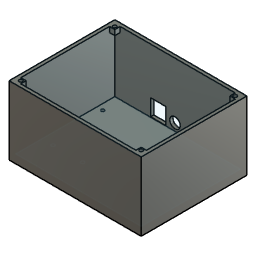
Arduino_Housing_v7 (Autodesk Fusion 360 design; units mm, degrees)
Autodesk Fusion 360 part; units mm, degrees
sketch "Sketch1" plane through (0, 0, 0) normal (0, 1, 0) x (1, 0, 0)
  line L0 (0, 0) -> (125, 0)
  line L1 (125, 0) -> (125, -100)
  line L2 (125, -100) -> (0, -100)
  line L3 (0, -100) -> (0, 0)
  dimension "d1" = 125
  dimension "d2" = 100
  constraint horizontal L0
  constraint vertical L1
  constraint horizontal L2
  constraint vertical L3
  constraint coincident L0.start L3.end
  measures "d1" distance of L0.start L0.end
  measures "d2" distance of L0.start L2.end
extrude "Extrude1" add sketch "Sketch1" along normal blind 5
sketch "Sketch2" plane through (0, 5, 0) normal (0, 1, 0) x (-1, 0, 0)
  line L0 (0, 100) -> (-125, 100)
  line L1 (-125, 100) -> (-125, 0)
  line L2 (-125, 0) -> (0, 0)
  line L3 (0, 0) -> (0, 100)
  line L4 (-122, 3) -> (-3, 3)
  line L5 (-3, 3) -> (-3, 97)
  line L6 (-3, 97) -> (-122, 97)
  line L7 (-122, 97) -> (-122, 3)
  line L8 (-6, 6) -> (-59.3, 6)
  line L9 (-59.3, 6) -> (-59.3, 74.6)
  line L10 (-59.3, 74.6) -> (-6, 74.6)
  line L11 (-6, 74.6) -> (-6, 6)
  line L12 (-59.3, 6) -> (-52.3, 6)
  line L13 (-6, 6) -> (-37, 6)
  line L14 (-37, 3) -> (-52, 3)
  line L15 (-52, 3) -> (-52, 0)
  line L16 (-52, 0) -> (-37, 0)
  line L17 (-37, 0) -> (-37, 3)
  line L18 (-6, 6) -> (-6, 19.97)
  circle A0 centre (-8.54, 19.97) radius 1.5
  line L19 (-6, 6) -> (-6, 72.04)
  circle A1 centre (-13.62, 72.04) radius 1.65
  circle A2 centre (-41.56, 72.04) radius 1.65
  line L20 (-119, 6) -> (-64, 6)
  line L21 (-64, 6) -> (-64, 90)
  line L22 (-64, 90) -> (-119, 90)
  line L23 (-119, 90) -> (-119, 6)
  dimension "d9" = 53.3
  dimension "d10" = 68.6
  dimension "d11" = 7
  dimension "d12" = 31
  dimension "d13" = 13.97
  dimension "d14" = 2.54
  dimension "d15" = 3
  dimension "d16" = 66.04
  dimension "d17" = 7.62
  dimension "d18" = 35.56
  dimension "d19" = 3.3
  dimension "d20" = 3.3
  dimension "d21" = 55
  dimension "d22" = 84
  constraint horizontal L4
  constraint vertical L5
  constraint horizontal L6
  constraint vertical L7
  constraint horizontal L8
  constraint vertical L9
  constraint horizontal L10
  constraint vertical L11
  constraint perpendicular L9 L12
  constraint perpendicular L11 L13
  constraint horizontal L14
  constraint vertical L15
  constraint horizontal L16
  constraint vertical L17
  constraint coincident L2 L15.end
  constraint coincident L4 L14.start
  constraint perpendicular L13 L18
  constraint perpendicular L13 L19
  constraint horizontal L20
  constraint vertical L21
  constraint horizontal L22
  constraint vertical L23
  measures "d9" distance of L8.start L8.end
  measures "d10" distance of L8.start L10.end
  measures "d11" distance of L8.end L12.end
  measures "d12" distance of L8.start L13.end
  measures "d13" distance of L8.start L18.end
  measures "d14" distance of L18.end A0.centre
  measures "d15" diameter of A0
  measures "d16" distance of L8.start L19.end
  measures "d17" distance of L19.end A1.centre
  measures "d18" distance of L19.end A2.centre
  measures "d19" diameter of A1
  measures "d20" diameter of A2
  measures "d21" distance of L20.start L20.end
  measures "d22" distance of L20.start L22.end
extrude "Extrude2" cut sketch "Sketch2" against normal blind 5 contours A0 | A1 | A2
sketch "Sketch3" plane through (0, 5, 0) normal (0, 1, 0) x (-1, 0, 0)
  circle A0 centre (-8.54, 19.97) radius 1.5
  circle A1 centre (-13.62, 72.04) radius 1.65
  circle A2 centre (-41.56, 72.04) radius 1.65
  line L0 (0, 100) -> (-125, 100)
  line L1 (-125, 100) -> (-125, 0)
  line L2 (-125, 0) -> (0, 0)
  line L3 (0, 0) -> (0, 100)
  line L4 (-3, 3) -> (-123.5, 3)
  line L5 (-123.5, 3) -> (-123.5, 98.5)
  line L6 (-123.5, 98.5) -> (-3, 98.5)
  line L7 (-3, 98.5) -> (-3, 3)
  line L8 (-6, 6) -> (-59.3, 6)
  line L9 (-59.3, 6) -> (-59.3, 74.6)
  line L10 (-59.3, 74.6) -> (-6, 74.6)
  line L11 (-6, 74.6) -> (-6, 6)
  line L12 (-6, 6) -> (-37, 6)
  line L13 (-59.3, 6) -> (-51.3, 6)
  line L14 (-37, 3) -> (-51.3, 3)
  line L15 (-51.3, 3) -> (-51.3, 0)
  line L16 (-51.3, 0) -> (-37, 0)
  line L17 (-37, 0) -> (-37, 3)
  dimension "d25" = 53.3
  dimension "d26" = 68.6
  dimension "d27" = 31
  dimension "d28" = 8
  constraint horizontal L4
  constraint vertical L5
  constraint horizontal L6
  constraint vertical L7
  constraint horizontal L8
  constraint vertical L9
  constraint horizontal L10
  constraint vertical L11
  constraint perpendicular L11 L12
  constraint perpendicular L9 L13
  constraint horizontal L14
  constraint vertical L15
  constraint horizontal L16
  constraint vertical L17
  constraint coincident L2 L15.end
  constraint coincident L4 L14.start
  measures "d25" distance of L8.start L8.end
  measures "d26" distance of L8.start L10.end
  measures "d27" distance of L8.start L12.end
  measures "d28" distance of L8.end L13.end
extrude "Extrude3" add sketch "Sketch3" along normal blind 1 contours L0 L1 L2 L3 L4 L5 L6 L7 L15 L17
sketch "Sketch4" plane through (0, 0, 0) normal (0, -1, 0) x (1, 0, 0)
  circle A0 centre (8.54, 19.97) radius 1.5
  circle A1 centre (13.62, 72.04) radius 1.65
  circle A2 centre (41.56, 72.04) radius 1.65
  line L0 (125, 100) -> (0, 100)
  line L1 (0, 100) -> (0, 0)
  line L2 (0, 0) -> (125, 0)
  line L3 (125, 0) -> (125, 100)
  circle A3 centre (8.54, 19.97) radius 3.5
  circle A4 centre (13.62, 72.04) radius 3.5
  circle A5 centre (41.56, 72.04) radius 3.5
  dimension "d31" = 7
  dimension "d32" = 7
  dimension "d33" = 7
  constraint concentric A0 A3
  constraint concentric A1 A4
  constraint concentric A2 A5
  measures "d31" diameter of A3
  measures "d32" diameter of A4
  measures "d33" diameter of A5
extrude "Extrude4" cut sketch "Sketch4" against normal blind 2.5 contours A3 | A4 | A5
extrude "Extrude5" add 1 faces at (1, 6, 34.3333) along direction (0, 1, 0) blind 17
sketch "Sketch5" plane through (0, 5, 0) normal (0, 1, 0) x (-1, 0, 0)
  line L0 (-51.3, 3) -> (-51.3, 0)
  line L1 (-51.3, 0) -> (-37, 0)
  line L2 (-37, 0) -> (-37, 3)
  line L3 (-37, 3) -> (-3, 3)
  line L4 (-3, 3) -> (-3, 98.5)
  line L5 (-3, 98.5) -> (-123.5, 98.5)
  line L6 (-123.5, 98.5) -> (-123.5, 3)
  line L7 (-123.5, 3) -> (-51.3, 3)
  circle A0 centre (-8.54, 19.97) radius 1.5
  circle A1 centre (-13.62, 72.04) radius 1.65
  circle A2 centre (-41.56, 72.04) radius 1.65
  line L8 (-51.3, 3) -> (-37, 3)
  line L9 (-37, 3) -> (-37, 0)
  line L10 (-37, 0) -> (-51.3, 0)
  line L11 (-51.3, 0) -> (-51.3, 3)
  constraint horizontal L8
  constraint vertical L9
  constraint horizontal L10
  constraint vertical L11
  constraint coincident L1.end L2.start
  constraint coincident L0.start L7.end
extrude "Extrude6" add sketch "Sketch5" along normal blind 0.4 contours L0 L1 L2 L8 L9 L10 L11
extrude "Extrude7" cut 1 faces at (1, 23, 34.3333) along direction (0, -1, 0) blind 2
sketch "Sketch6" plane through (0, 21, 0) normal (0, 1, 0) x (-1, 0, 0)
  line L0 (0, 0) -> (0, 100)
  line L1 (0, 100) -> (-125, 100)
  line L2 (-125, 100) -> (-125, 0)
  line L3 (-125, 0) -> (-51.3, 0)
  line L4 (-51.3, 0) -> (-51.3, 3)
  line L5 (-51.3, 3) -> (-123.5, 3)
  line L6 (-123.5, 3) -> (-123.5, 98.5)
  line L7 (-123.5, 98.5) -> (-3, 98.5)
  line L8 (-3, 98.5) -> (-3, 3)
  line L9 (-3, 3) -> (-37, 3)
  line L10 (-37, 3) -> (-37, 0)
  line L11 (-37, 0) -> (0, 0)
  line L12 (-37, 0) -> (-51.3, 0)
  line L13 (-51.3, 0) -> (-51.3, 3)
  line L14 (-51.3, 3) -> (-37, 3)
  line L15 (-37, 3) -> (-37, 0)
  constraint horizontal L12
  constraint vertical L13
  constraint horizontal L14
  constraint vertical L15
  constraint coincident L4.end L5.start
  constraint coincident L10.end L11.start
extrude "Extrude8" add sketch "Sketch6" along normal blind 44 contours L0 L1 L2 L3 L4 L5 L6 L7 L8 L9 L10 L11 L13 L15 | L4 L10 L12 L13 L14 L15
sketch "Sketch7" plane through (0, 0, 3) normal (0, 0, 1) x (1, 0, 0)
  line L0 (3, 65) -> (3, 5)
  line L1 (3, 5) -> (123.5, 5)
  line L2 (123.5, 5) -> (123.5, 65)
  line L3 (123.5, 65) -> (3, 65)
  line L4 (37, 21) -> (51.3, 21)
  line L5 (51.3, 21) -> (51.3, 5.4)
  line L6 (51.3, 5.4) -> (37, 5.4)
  line L7 (37, 5.4) -> (37, 21)
  circle A0 centre (60, 12) radius 5
  dimension "d44" = 10
  measures "d44" diameter of A0
extrude "Extrude9" cut sketch "Sketch7" against normal blind 3 contours A0
extrude "Extrude10" add 1 faces at (43.1667, 45, 98.5) along direction (0, 0, -1) blind 1.5
extrude "Extrude11" add 1 faces at (123.5, 25, 34.3333) along direction (-1, 0, 0) blind 1.5
sketch "Sketch8" plane through (0, 5, 0) normal (0, 1, 0) x (-1, 0, 0)
  line L0 (-122, 97) -> (-122, 3)
  line L1 (-122, 3) -> (-3, 3)
  line L2 (-3, 3) -> (-3, 97)
  line L3 (-3, 97) -> (-122, 97)
  circle A0 centre (-41.56, 72.04) radius 1.65
  circle A1 centre (-13.62, 72.04) radius 1.65
  circle A2 centre (-8.54, 19.97) radius 1.5
sketch "Sketch9" plane through (0, 65, 0) normal (0, 1, 0) x (-1, 0, 0)
  line L0 (-3, 3) -> (-122, 3)
  line L1 (-122, 3) -> (-122, 97)
  line L2 (-122, 97) -> (-3, 97)
  line L3 (-3, 97) -> (-3, 3)
  line L4 (0, 0) -> (0, 100)
  line L5 (0, 100) -> (-125, 100)
  line L6 (-125, 100) -> (-125, 0)
  line L7 (-125, 0) -> (0, 0)
  line L8 (-122, 97) -> (-112, 97)
  line L9 (-112, 97) -> (-112, 87)
  line L10 (-112, 87) -> (-122, 87)
  line L11 (-122, 87) -> (-122, 97)
  line L12 (-122, 3) -> (-112, 3)
  line L13 (-112, 3) -> (-112, 13)
  line L14 (-112, 13) -> (-122, 13)
  line L15 (-122, 13) -> (-122, 3)
  line L16 (-3, 97) -> (-13, 97)
  line L17 (-13, 97) -> (-13, 87)
  line L18 (-13, 87) -> (-3, 87)
  line L19 (-3, 87) -> (-3, 97)
  line L20 (-3, 3) -> (-13, 3)
  line L21 (-13, 3) -> (-13, 13)
  line L22 (-13, 13) -> (-3, 13)
  line L23 (-3, 13) -> (-3, 3)
  dimension "d51" = 10
  dimension "d52" = 10
  dimension "d53" = 10
  dimension "d54" = 10
  dimension "d55" = 10
  dimension "d56" = 10
  constraint horizontal L8
  constraint vertical L9
  constraint horizontal L10
  constraint vertical L11
  constraint coincident L1.end L2.start
  constraint horizontal L12
  constraint vertical L13
  constraint horizontal L14
  constraint vertical L15
  constraint coincident L0.end L1.start
  constraint horizontal L16
  constraint vertical L17
  constraint horizontal L18
  constraint vertical L19
  constraint coincident L2.end L3.start
  constraint horizontal L20
  constraint vertical L21
  constraint horizontal L22
  constraint vertical L23
  constraint coincident L0.start L3.end
  measures "d51" distance of L0.end L12.end
  measures "d52" distance of L0.end L14.end
  measures "d53" distance of L2.end L16.end
  measures "d54" distance of L2.end L18.end
  measures "d55" distance of L0.start L20.end
  measures "d56" distance of L0.start L22.end
extrude "Extrude12" add sketch "Sketch9" against normal blind 3 contours L0 L3 L20 L21 L22 L23 | L0 L1 L12 L13 L14 L15 | L2 L3 L16 L17 L18 L19 | L1 L2 L8 L9 L10 L11
sketch "Sketch10" plane through (0, 65, 0) normal (0, 1, 0) x (-1, 0, 0)
  line L0 (-13, 3) -> (-112, 3)
  line L1 (-112, 3) -> (-112, 13)
  line L2 (-112, 13) -> (-122, 13)
  line L3 (-122, 13) -> (-122, 87)
  line L4 (-122, 87) -> (-112, 87)
  line L5 (-112, 87) -> (-112, 97)
  line L6 (-112, 97) -> (-13, 97)
  line L7 (-13, 97) -> (-13, 87)
  line L8 (-13, 87) -> (-3, 87)
  line L9 (-3, 87) -> (-3, 13)
  line L10 (-3, 13) -> (-13, 13)
  line L11 (-13, 13) -> (-13, 3)
  line L12 (0, 0) -> (0, 100)
  line L13 (0, 100) -> (-125, 100)
  line L14 (-125, 100) -> (-125, 0)
  line L15 (-125, 0) -> (0, 0)
  circle A0 centre (-8, 8) radius 1.65
  circle A1 centre (-8, 92) radius 1.65
  circle A2 centre (-117, 92) radius 1.65
  circle A3 centre (-117, 8) radius 1.65
  dimension "d59" = 3.3
  dimension "d60" = 3.3
  dimension "d61" = 3.3
  dimension "d62" = 3.3
  measures "d59" diameter of A0
  measures "d60" diameter of A1
  measures "d61" diameter of A2
  measures "d62" diameter of A3
extrude "Extrude13" cut sketch "Sketch10" against normal blind 3 contours A0 | A1 | A2 | A3
delete_face "DeleteFace1" 1 faces at (115.3521, 63, 91.9178)
delete_face "DeleteFace2" 1 faces at (117.7527, 63, 6.5317)
delete_face "DeleteFace3" 2 faces at (6.3582, 64, 7.8357) (6.3521, 63, 91.9178)
sketch "Sketch11" plane through (0, 65, 0) normal (0, 1, 0) x (-1, 0, 0)
  line L0 (-13, 3) -> (-112, 3)
  line L1 (-112, 3) -> (-112, 13)
  line L2 (-112, 13) -> (-122, 13)
  line L3 (-122, 13) -> (-122, 87)
  line L4 (-122, 87) -> (-112, 87)
  line L5 (-112, 87) -> (-112, 97)
  line L6 (-112, 97) -> (-13, 97)
  line L7 (-13, 97) -> (-13, 87)
  line L8 (-13, 87) -> (-3, 87)
  line L9 (-3, 87) -> (-3, 13)
  line L10 (-3, 13) -> (-13, 13)
  line L11 (-13, 13) -> (-13, 3)
  line L12 (0, 0) -> (0, 100)
  line L13 (0, 100) -> (-125, 100)
  line L14 (-125, 100) -> (-125, 0)
  line L15 (-125, 0) -> (0, 0)
  line L16 (-13, 13) -> (-3, 13)
  line L17 (-3, 13) -> (-3, 3)
  line L18 (-3, 3) -> (-13, 3)
  line L19 (-13, 3) -> (-13, 13)
  line L20 (-13, 87) -> (-3, 87)
  line L21 (-3, 87) -> (-3, 97)
  line L22 (-3, 97) -> (-13, 97)
  line L23 (-13, 97) -> (-13, 87)
  line L24 (-112, 87) -> (-122, 87)
  line L25 (-122, 87) -> (-122, 97)
  line L26 (-122, 97) -> (-112, 97)
  line L27 (-112, 97) -> (-112, 87)
  line L28 (-112, 13) -> (-122, 13)
  line L29 (-122, 13) -> (-122, 3)
  line L30 (-122, 3) -> (-112, 3)
  line L31 (-112, 3) -> (-112, 13)
  constraint horizontal L16
  constraint vertical L17
  constraint horizontal L18
  constraint vertical L19
  constraint coincident L10.end L11.start
  constraint horizontal L20
  constraint vertical L21
  constraint horizontal L22
  constraint vertical L23
  constraint coincident L7.end L8.start
  constraint horizontal L24
  constraint vertical L25
  constraint horizontal L26
  constraint vertical L27
  constraint coincident L4.end L5.start
  constraint horizontal L28
  constraint vertical L29
  constraint horizontal L30
  constraint vertical L31
  constraint coincident L1.end L2.start
extrude "Extrude14" cut sketch "Sketch11" against normal blind 3 contours L10 L11 L16 L17 L18 L19 | L1 L2 L28 L29 L30 L31 | L7 L8 L20 L21 L22 L23 | L4 L5 L24 L25 L26 L27
sketch "Sketch12" plane through (0, 65, 0) normal (0, 1, 0) x (-1, 0, 0)
  line L0 (-3, 97) -> (-3, 3)
  line L1 (-3, 3) -> (-122, 3)
  line L2 (-122, 3) -> (-122, 97)
  line L3 (-122, 97) -> (-3, 97)
  line L4 (0, 0) -> (0, 100)
  line L5 (0, 100) -> (-125, 100)
  line L6 (-125, 100) -> (-125, 0)
  line L7 (-125, 0) -> (0, 0)
  line L8 (-3, 3) -> (-8, 3)
  line L9 (-8, 3) -> (-8, 8)
  line L10 (-8, 8) -> (-3, 8)
  line L11 (-3, 8) -> (-3, 3)
  line L12 (-3, 97) -> (-8, 97)
  line L13 (-8, 97) -> (-8, 92)
  line L14 (-8, 92) -> (-3, 92)
  line L15 (-3, 92) -> (-3, 97)
  line L16 (-122, 97) -> (-117, 97)
  line L17 (-117, 97) -> (-117, 92)
  line L18 (-117, 92) -> (-122, 92)
  line L19 (-122, 92) -> (-122, 97)
  line L20 (-122, 3) -> (-117, 3)
  line L21 (-117, 3) -> (-117, 8)
  line L22 (-117, 8) -> (-122, 8)
  line L23 (-122, 8) -> (-122, 3)
  constraint horizontal L8
  constraint vertical L9
  constraint horizontal L10
  constraint vertical L11
  constraint coincident L0.end L1.start
  constraint horizontal L12
  constraint vertical L13
  constraint horizontal L14
  constraint vertical L15
  constraint coincident L0.start L3.end
  constraint horizontal L16
  constraint vertical L17
  constraint horizontal L18
  constraint vertical L19
  constraint coincident L2.end L3.start
  constraint horizontal L20
  constraint vertical L21
  constraint horizontal L22
  constraint vertical L23
  constraint coincident L1.end L2.start
extrude "Extrude15" add sketch "Sketch12" against normal blind 5 contours L0 L3 L12 L13 L14 L15 | L0 L1 L8 L9 L10 L11 | L2 L3 L16 L17 L18 L19 | L1 L2 L20 L21 L22 L23
sketch "Sketch13" plane through (0, 65, 0) normal (0, 1, 0) x (-1, 0, 0)
  line L0 (-3, 92) -> (-3, 8)
  line L1 (-3, 8) -> (-8, 8)
  line L2 (-8, 8) -> (-8, 3)
  line L3 (-8, 3) -> (-117, 3)
  line L4 (-117, 3) -> (-117, 8)
  line L5 (-117, 8) -> (-122, 8)
  line L6 (-122, 8) -> (-122, 92)
  line L7 (-122, 92) -> (-117, 92)
  line L8 (-117, 92) -> (-117, 97)
  line L9 (-117, 97) -> (-8, 97)
  line L10 (-8, 97) -> (-8, 92)
  line L11 (-8, 92) -> (-3, 92)
  line L12 (0, 0) -> (0, 100)
  line L13 (0, 100) -> (-125, 100)
  line L14 (-125, 100) -> (-125, 0)
  line L15 (-125, 0) -> (0, 0)
  circle A0 centre (-5.5, 5.5) radius 1.65
  line L16 (-8, 92) -> (-5.5, 92)
  line L17 (-8, 94.5) -> (-8, 92)
  circle A1 centre (-5.5, 94.5) radius 1.65
  line L18 (-117, 92) -> (-119.5, 92)
  line L19 (-117, 94.5) -> (-117, 92)
  circle A2 centre (-119.5, 94.5) radius 1.65
  line L20 (-117, 8) -> (-119.5, 8)
  line L21 (-117, 5.5) -> (-117, 8)
  circle A3 centre (-119.5, 5.5) radius 1.65
  dimension "d69" = 3.3
  dimension "d70" = 3.3
  dimension "d71" = 3.3
  dimension "d72" = 3.3
  constraint horizontal L16
  constraint vertical L17
  constraint coincident L10.end L11.start
  constraint horizontal L18
  constraint vertical L19
  constraint coincident L7.end L8.start
  constraint horizontal L20
  constraint vertical L21
  constraint coincident L4.end L5.start
  measures "d69" diameter of A0
  measures "d70" diameter of A1
  measures "d71" diameter of A2
  measures "d72" diameter of A3
extrude "Extrude16" cut sketch "Sketch13" against normal blind 5 contours A0 | A1 | A2 | A3
sketch "Sketch14" plane through (0, 65, 0) normal (0, 1, 0) x (-1, 0, 0)
  circle A0 centre (-119.5, 5.5) radius 1.65
  circle A1 centre (-5.5, 5.5) radius 1.65
  circle A2 centre (-119.5, 94.5) radius 1.65
  circle A3 centre (-5.5, 94.5) radius 1.65
  line L0 (-3, 92) -> (-3, 8)
  line L1 (-3, 8) -> (-8, 8)
  line L2 (-8, 8) -> (-8, 3)
  line L3 (-8, 3) -> (-117, 3)
  line L4 (-117, 3) -> (-117, 8)
  line L5 (-117, 8) -> (-122, 8)
  line L6 (-122, 8) -> (-122, 92)
  line L7 (-122, 92) -> (-117, 92)
  line L8 (-117, 92) -> (-117, 97)
  line L9 (-117, 97) -> (-8, 97)
  line L10 (-8, 97) -> (-8, 92)
  line L11 (-8, 92) -> (-3, 92)
  line L12 (0, 0) -> (0, 100)
  line L13 (0, 100) -> (-125, 100)
  line L14 (-125, 100) -> (-125, 0)
  line L15 (-125, 0) -> (0, 0)
